Autodesk Inventor part; units mm, degrees
(part 2 of 2)
  line L647 (139.4375, -211.0124) -> (136.5507, -216.0124)
  line L648 (136.5507, -221.0124) -> (139.4375, -226.0124)
  line L649 (139.4375, -226.0124) -> (136.5507, -231.0124)
  line L650 (130.7772, -221.0124) -> (136.5507, -221.0124)
  line L651 (136.5507, -231.0124) -> (130.7772, -231.0124)
  line L652 (130.7772, -231.0124) -> (127.8905, -226.0124)
  line L653 (127.8905, -226.0124) -> (130.7772, -221.0124)
  line L654 (136.5507, -206.0124) -> (139.4375, -211.0124)
  line L655 (136.5507, -216.0124) -> (130.7772, -216.0124)
  line L656 (130.7772, -216.0124) -> (127.8905, -211.0124)
  line L657 (130.7772, -206.0124) -> (136.5507, -206.0124)
  line L658 (127.8905, -211.0124) -> (130.7772, -206.0124)
  line L659 (140.8809, -218.5124) -> (143.7676, -213.5124)
  line L660 (143.7676, -213.5124) -> (149.5411, -213.5124)
  line L661 (149.5411, -213.5124) -> (152.4279, -218.5124)
  line L662 (149.5411, -223.5124) -> (143.7676, -223.5124)
  line L663 (152.4279, -218.5124) -> (149.5411, -223.5124)
  line L664 (143.7676, -223.5124) -> (140.8809, -218.5124)
  line L665 (139.4375, -181.0124) -> (136.5507, -186.0124)
  line L666 (130.7772, -186.0124) -> (127.8905, -181.0124)
  line L667 (136.5507, -186.0124) -> (130.7772, -186.0124)
  line L668 (136.5507, -191.0124) -> (139.4375, -196.0124)
  line L669 (127.8905, -196.0124) -> (130.7772, -191.0124)
  line L670 (139.4375, -196.0124) -> (136.5507, -201.0124)
  line L671 (130.7772, -201.0124) -> (127.8905, -196.0124)
  line L672 (136.5507, -201.0124) -> (130.7772, -201.0124)
  line L673 (130.7772, -191.0124) -> (136.5507, -191.0124)
  line L674 (152.4279, -203.5124) -> (149.5411, -208.5124)
  line L675 (149.5411, -198.5124) -> (152.4279, -203.5124)
  line L676 (162.5507, -176.0124) -> (165.4375, -181.0124)
  line L677 (156.7772, -176.0124) -> (162.5507, -176.0124)
  line L678 (153.8905, -181.0124) -> (156.7772, -176.0124)
  line L679 (175.5411, -208.5124) -> (169.7676, -208.5124)
  line L680 (169.7676, -198.5124) -> (175.5411, -198.5124)
  line L681 (178.4279, -188.5124) -> (175.5411, -193.5124)
  line L682 (175.5411, -193.5124) -> (169.7676, -193.5124)
  line L683 (175.5411, -183.5124) -> (178.4279, -188.5124)
  line L684 (169.7676, -183.5124) -> (175.5411, -183.5124)
  line L685 (169.7676, -208.5124) -> (166.8809, -203.5124)
  line L686 (166.8809, -203.5124) -> (169.7676, -198.5124)
  line L687 (169.7676, -193.5124) -> (166.8809, -188.5124)
  line L688 (166.8809, -188.5124) -> (169.7676, -183.5124)
  line L689 (165.4375, -211.0124) -> (162.5507, -216.0124)
  line L690 (162.5507, -221.0124) -> (165.4375, -226.0124)
  line L691 (165.4375, -226.0124) -> (162.5507, -231.0124)
  line L692 (156.7772, -221.0124) -> (162.5507, -221.0124)
  line L693 (162.5507, -231.0124) -> (156.7772, -231.0124)
  line L694 (156.7772, -231.0124) -> (153.8905, -226.0124)
  line L695 (153.8905, -226.0124) -> (156.7772, -221.0124)
  line L696 (162.5507, -206.0124) -> (165.4375, -211.0124)
  line L697 (162.5507, -216.0124) -> (156.7772, -216.0124)
  line L698 (156.7772, -216.0124) -> (153.8905, -211.0124)
  line L699 (156.7772, -206.0124) -> (162.5507, -206.0124)
  line L700 (153.8905, -211.0124) -> (156.7772, -206.0124)
  line L701 (166.8809, -218.5124) -> (169.7676, -213.5124)
  line L702 (169.7676, -213.5124) -> (175.5411, -213.5124)
  line L703 (175.5411, -213.5124) -> (178.4279, -218.5124)
  line L704 (175.5411, -223.5124) -> (169.7676, -223.5124)
  line L705 (178.4279, -218.5124) -> (175.5411, -223.5124)
  line L706 (169.7676, -223.5124) -> (166.8809, -218.5124)
  line L707 (165.4375, -181.0124) -> (162.5507, -186.0124)
  line L708 (156.7772, -186.0124) -> (153.8905, -181.0124)
  line L709 (162.5507, -186.0124) -> (156.7772, -186.0124)
  line L710 (162.5507, -191.0124) -> (165.4375, -196.0124)
  line L711 (153.8905, -196.0124) -> (156.7772, -191.0124)
  line L712 (165.4375, -196.0124) -> (162.5507, -201.0124)
  line L713 (156.7772, -201.0124) -> (153.8905, -196.0124)
  line L714 (162.5507, -201.0124) -> (156.7772, -201.0124)
  line L715 (156.7772, -191.0124) -> (162.5507, -191.0124)
  line L716 (178.4279, -203.5124) -> (175.5411, -208.5124)
  line L717 (175.5411, -198.5124) -> (178.4279, -203.5124)
  line L718 (188.5507, -176.0124) -> (191.4375, -181.0124)
  line L719 (182.7772, -176.0124) -> (188.5507, -176.0124)
  line L720 (179.8905, -181.0124) -> (182.7772, -176.0124)
  line L721 (201.5411, -208.5124) -> (195.7676, -208.5124)
  line L722 (195.7676, -198.5124) -> (201.5411, -198.5124)
  line L723 (204.4279, -188.5124) -> (201.5411, -193.5124)
  line L724 (201.5411, -193.5124) -> (195.7676, -193.5124)
  line L725 (201.5411, -183.5124) -> (204.4279, -188.5124)
  line L726 (195.7676, -183.5124) -> (201.5411, -183.5124)
  line L727 (195.7676, -208.5124) -> (192.8809, -203.5124)
  line L728 (192.8809, -203.5124) -> (195.7676, -198.5124)
  line L729 (195.7676, -193.5124) -> (192.8809, -188.5124)
  line L730 (192.8809, -188.5124) -> (195.7676, -183.5124)
  line L731 (191.4375, -211.0124) -> (188.5507, -216.0124)
  line L732 (188.5507, -221.0124) -> (191.4375, -226.0124)
  line L733 (191.4375, -226.0124) -> (188.5507, -231.0124)
  line L734 (182.7772, -221.0124) -> (188.5507, -221.0124)
  line L735 (188.5507, -231.0124) -> (182.7772, -231.0124)
  line L736 (182.7772, -231.0124) -> (179.8905, -226.0124)
  line L737 (179.8905, -226.0124) -> (182.7772, -221.0124)
  line L738 (188.5507, -206.0124) -> (191.4375, -211.0124)
  line L739 (188.5507, -216.0124) -> (182.7772, -216.0124)
  line L740 (182.7772, -216.0124) -> (179.8905, -211.0124)
  line L741 (182.7772, -206.0124) -> (188.5507, -206.0124)
  line L742 (179.8905, -211.0124) -> (182.7772, -206.0124)
  line L743 (192.8809, -218.5124) -> (195.7676, -213.5124)
  line L744 (195.7676, -213.5124) -> (201.5411, -213.5124)
  line L745 (201.5411, -213.5124) -> (204.4279, -218.5124)
  line L746 (201.5411, -223.5124) -> (195.7676, -223.5124)
  line L747 (204.4279, -218.5124) -> (201.5411, -223.5124)
  line L748 (195.7676, -223.5124) -> (192.8809, -218.5124)
  line L749 (191.4375, -181.0124) -> (188.5507, -186.0124)
  line L750 (182.7772, -186.0124) -> (179.8905, -181.0124)
  line L751 (188.5507, -186.0124) -> (182.7772, -186.0124)
  line L752 (188.5507, -191.0124) -> (191.4375, -196.0124)
  line L753 (179.8905, -196.0124) -> (182.7772, -191.0124)
  line L754 (191.4375, -196.0124) -> (188.5507, -201.0124)
  line L755 (182.7772, -201.0124) -> (179.8905, -196.0124)
  line L756 (188.5507, -201.0124) -> (182.7772, -201.0124)
  line L757 (182.7772, -191.0124) -> (188.5507, -191.0124)
  line L758 (204.4279, -203.5124) -> (201.5411, -208.5124)
  line L759 (201.5411, -198.5124) -> (204.4279, -203.5124)
  line L760 (214.5507, -176.0124) -> (217.4375, -181.0124)
  line L761 (208.7772, -176.0124) -> (214.5507, -176.0124)
  line L762 (205.8905, -181.0124) -> (208.7772, -176.0124)
  line L763 (227.5411, -208.5124) -> (221.7676, -208.5124)
  line L764 (221.7676, -198.5124) -> (227.5411, -198.5124)
  line L765 (230.4279, -188.5124) -> (227.5411, -193.5124)
  line L766 (227.5411, -193.5124) -> (221.7676, -193.5124)
  line L767 (227.5411, -183.5124) -> (230.4279, -188.5124)
  line L768 (221.7676, -183.5124) -> (227.5411, -183.5124)
  line L769 (221.7676, -208.5124) -> (218.8809, -203.5124)
  line L770 (218.8809, -203.5124) -> (221.7676, -198.5124)
  line L771 (221.7676, -193.5124) -> (218.8809, -188.5124)
  line L772 (218.8809, -188.5124) -> (221.7676, -183.5124)
  line L773 (217.4375, -211.0124) -> (214.5507, -216.0124)
  line L774 (214.5507, -221.0124) -> (217.4375, -226.0124)
  line L775 (217.4375, -226.0124) -> (214.5507, -231.0124)
  line L776 (208.7772, -221.0124) -> (214.5507, -221.0124)
  line L777 (214.5507, -231.0124) -> (208.7772, -231.0124)
  line L778 (208.7772, -231.0124) -> (205.8905, -226.0124)
  line L779 (205.8905, -226.0124) -> (208.7772, -221.0124)
  line L780 (214.5507, -206.0124) -> (217.4375, -211.0124)
  line L781 (214.5507, -216.0124) -> (208.7772, -216.0124)
  line L782 (208.7772, -216.0124) -> (205.8905, -211.0124)
  line L783 (208.7772, -206.0124) -> (214.5507, -206.0124)
  line L784 (205.8905, -211.0124) -> (208.7772, -206.0124)
  line L785 (218.8809, -218.5124) -> (221.7676, -213.5124)
  line L786 (221.7676, -213.5124) -> (227.5411, -213.5124)
  line L787 (227.5411, -213.5124) -> (230.4279, -218.5124)
  line L788 (227.5411, -223.5124) -> (221.7676, -223.5124)
  line L789 (230.4279, -218.5124) -> (227.5411, -223.5124)
  line L790 (221.7676, -223.5124) -> (218.8809, -218.5124)
  line L791 (217.4375, -181.0124) -> (214.5507, -186.0124)
  line L792 (208.7772, -186.0124) -> (205.8905, -181.0124)
  line L793 (214.5507, -186.0124) -> (208.7772, -186.0124)
  line L794 (214.5507, -191.0124) -> (217.4375, -196.0124)
  line L795 (205.8905, -196.0124) -> (208.7772, -191.0124)
  line L796 (217.4375, -196.0124) -> (214.5507, -201.0124)
  line L797 (208.7772, -201.0124) -> (205.8905, -196.0124)
  line L798 (214.5507, -201.0124) -> (208.7772, -201.0124)
  line L799 (208.7772, -191.0124) -> (214.5507, -191.0124)
  line L800 (230.4279, -203.5124) -> (227.5411, -208.5124)
  line L801 (227.5411, -198.5124) -> (230.4279, -203.5124)
  point P0 (0, 0)
  point P1 (-256.336, -226.0124)
  point P2 (-243.3456, -218.5124)
  point P3 (-256.336, -211.0124)
  point P4 (-243.3456, -203.5124)
  point P5 (-256.336, -196.0124)
  point P6 (-243.3456, -188.5124)
  point P7 (-256.336, -181.0124)
  point P8 (-217.3456, -203.5124)
  point P9 (-217.3456, -188.5124)
  point P10 (-230.336, -226.0124)
  point P11 (-230.336, -211.0124)
  point P12 (-217.3456, -218.5124)
  point P13 (-230.336, -181.0124)
  point P14 (-230.336, -196.0124)
  point P15 (-191.3456, -203.5124)
  point P16 (-191.3456, -188.5124)
  point P17 (-204.336, -226.0124)
  point P18 (-204.336, -211.0124)
  point P19 (-191.3456, -218.5124)
  point P20 (-204.336, -181.0124)
  point P21 (-204.336, -196.0124)
  point P22 (-165.3456, -203.5124)
  point P23 (-165.3456, -188.5124)
  point P24 (-178.336, -226.0124)
  point P25 (-178.336, -211.0124)
  point P26 (-165.3456, -218.5124)
  point P27 (-178.336, -181.0124)
  point P28 (-178.336, -196.0124)
  point P29 (-139.3456, -203.5124)
  point P30 (-139.3456, -188.5124)
  point P31 (-152.336, -226.0124)
  point P32 (-152.336, -211.0124)
  point P33 (-139.3456, -218.5124)
  point P34 (-152.336, -181.0124)
  point P35 (-152.336, -196.0124)
  point P36 (-113.3456, -203.5124)
  point P37 (-113.3456, -188.5124)
  point P38 (-126.336, -226.0124)
  point P39 (-126.336, -211.0124)
  point P40 (-113.3456, -218.5124)
  point P41 (-126.336, -181.0124)
  point P42 (-126.336, -196.0124)
  point P43 (-87.3456, -203.5124)
  point P44 (-87.3456, -188.5124)
  point P45 (-100.336, -226.0124)
  point P46 (-100.336, -211.0124)
  point P47 (-87.3456, -218.5124)
  point P48 (-100.336, -181.0124)
  point P49 (-100.336, -196.0124)
  point P50 (-61.3456, -203.5124)
  point P51 (-61.3456, -188.5124)
  point P52 (-74.336, -226.0124)
  point P53 (-74.336, -211.0124)
  point P54 (-61.3456, -218.5124)
  point P55 (-74.336, -181.0124)
  point P56 (-74.336, -196.0124)
  point P57 (-35.3456, -203.5124)
  point P58 (-35.3456, -188.5124)
  point P59 (-48.336, -226.0124)
  point P60 (-48.336, -211.0124)
  point P61 (-35.3456, -218.5124)
  point P62 (-48.336, -181.0124)
  point P63 (-48.336, -196.0124)
  point P64 (-9.3456, -203.5124)
  point P65 (-9.3456, -188.5124)
  point P66 (-22.336, -226.0124)
  point P67 (-22.336, -211.0124)
  point P68 (-9.3456, -218.5124)
  point P69 (-22.336, -181.0124)
  point P70 (-22.336, -196.0124)
  point P71 (16.6544, -203.5124)
  point P72 (16.6544, -188.5124)
  point P73 (3.664, -226.0124)
  point P74 (3.664, -211.0124)
  point P75 (16.6544, -218.5124)
  point P76 (3.664, -181.0124)
  point P77 (3.664, -196.0124)
  point P78 (42.6544, -203.5124)
  point P79 (42.6544, -188.5124)
  point P80 (29.664, -226.0124)
  point P81 (29.664, -211.0124)
  point P82 (42.6544, -218.5124)
  point P83 (29.664, -181.0124)
  point P84 (29.664, -196.0124)
  point P85 (68.6544, -203.5124)
  point P86 (68.6544, -188.5124)
  point P87 (55.664, -226.0124)
  point P88 (55.664, -211.0124)
  point P89 (68.6544, -218.5124)
  point P90 (55.664, -181.0124)
  point P91 (55.664, -196.0124)
  point P92 (94.6544, -203.5124)
  point P93 (94.6544, -188.5124)
  point P94 (81.664, -226.0124)
  point P95 (81.664, -211.0124)
  point P96 (94.6544, -218.5124)
  point P97 (81.664, -181.0124)
  point P98 (81.664, -196.0124)
  point P99 (120.6544, -203.5124)
  point P100 (120.6544, -188.5124)
  point P101 (107.664, -226.0124)
  point P102 (107.664, -211.0124)
  point P103 (120.6544, -218.5124)
  point P104 (107.664, -181.0124)
  point P105 (107.664, -196.0124)
  point P106 (146.6544, -203.5124)
  point P107 (146.6544, -188.5124)
  point P108 (133.664, -226.0124)
  point P109 (133.664, -211.0124)
  point P110 (146.6544, -218.5124)
  point P111 (133.664, -181.0124)
  point P112 (133.664, -196.0124)
  point P113 (172.6544, -203.5124)
  point P114 (172.6544, -188.5124)
  point P115 (159.664, -226.0124)
  point P116 (159.664, -211.0124)
  point P117 (172.6544, -218.5124)
  point P118 (159.664, -181.0124)
  point P119 (159.664, -196.0124)
  point P120 (198.6544, -203.5124)
  point P121 (198.6544, -188.5124)
  point P122 (185.664, -226.0124)
  point P123 (185.664, -211.0124)
  point P124 (198.6544, -218.5124)
  point P125 (185.664, -181.0124)
  point P126 (185.664, -196.0124)
  point P127 (224.6544, -203.5124)
  point P128 (224.6544, -188.5124)
  point P129 (211.664, -226.0124)
  point P130 (211.664, -211.0124)
  point P131 (224.6544, -218.5124)
  point P132 (211.664, -181.0124)
  point P133 (211.664, -196.0124)
  dimension "d39" = 10
  dimension "d40" = 22
  dimension "d41" = 5
  dimension "d42" = 5
  dimension "d43" = 5
  dimension "d46" = 15
  dimension "d53" = 26
  constraints: 1596 end point, 4 horizontal, 2 parallel, 2 vertical alignment, 1 vertical, 1729 other
  measures "d39" distance between parallel lines of L5 L8
  measures "d40" distance between parallel lines of L2 L5
  measures "d41" distance between parallel lines of L10 L9
  measures "d42" distance between parallel lines of L8 L16
  measures "d43" distance between parallel lines of L21 L11
  measures "d46" distance of L10.end L23.start
  measures "d53" distance of L38.start L46.start
equation "\"d2\" = d1"
equation "\"d8\" = d7"
equation "\"d10\" = d9"
equation "\"d11\" = d4"
equation "\"d42\" = d41"
equation "\"d43\" = d41"
equation "\"d9\" = d4"
body "Solid1"
